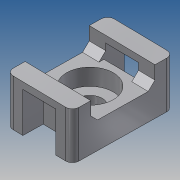
# Autodesk Inventor part: Příchytka pásků, pro M3, přírodní bílá
Saved by Autodesk Inventor 2020.4 (Build 244396000, 396)
## iProperties
Created: 2021-11-17
Part Number: Příchytka pásků, pro M3, přírodní bílá
Material: Plast, neprůhledný bílý
Catalog Web Link: https://www.plastovesoucastky.cz/cs/c/prichytky-pasku/prichytky-pasku-116?rozmerA=3.4
Vendor: plastovesoucastky
Document SubType Name: Modeling
Designer: Jiří Kizek
Manufacturer: Standard
Standards Organization: Custom
Mass: 0.453772 g
Surface Area: 7.13317 cm^2
Volume: 0.476652 cm^3
Density: 0.952 g/cm^3
Appearance: Hladká – bílá
Title: Příchytka pásků, pro M3, přírodní bílá
Author: Jiří Kizek
Keywords: 116 0004 000 02
QRDstProp: ███████ █████ ███████ █     █ █ █ █ █     █ █ ███ █ █     █ ███ █ █ ███ █ ████  █ ███ █ █ ███ █     █ █ ███ █ █     █ ██ █  █     █ ███████ █ █ █ ███████          ████         ██  ███  █ █   █ ████ █ █ ██ █   ██  █ █ ██  ██   ███ ██  █████   ██  ██ █ ██  ██ █ █   ██████████  ███   ██          ██  ███   ███ ███████  ██ ██     ██ █     █ █  ██  █ █    █ ███ █ ██ █  ███████ █ ███ █    ██  █ █ ██ █ ███ █   ██  █████   █     █ █    ██ █ █ █ ███████ ██  ███   ███
QRSrcProp: =<Part number> <Revision Number>
Povrch: 7,1331712703259
Hmotnost: 0,453772439604439
ProduktSkupina: 530
Autodesk Inventor part; units mm, degrees
ref_plane "YZ Plane" through (0, 0, 0) normal (1, 0, 0) x (0, 1, 0)
ref_plane "XZ Plane" through (0, 0, 0) normal (0, 1, 0) x (-1, 0, 0)
ref_plane "XY Plane" through (0, 0, 0) normal (0, 0, 1) x (1, 0, 0)
sketch "Náčrt6" plane through (0, 0, 0) normal (0, 1, 0) x (-1, 0, 0)
  line L0 (-7.5, 5) -> (7.5, 5)
  line L1 (7.5, 5) -> (7.5, -5)
  line L2 (7.5, -5) -> (-7.5, -5)
  line L3 (-7.5, -5) -> (-7.5, 5)
  line L4 (-7.5, 5) -> (7.5, -5) construction
  line L5 (7.5, 5) -> (-7.5, -5) construction
  point P0 (0, 0)
  dimension "d10" = 15
  dimension "d11" = 10
  constraints: 12 end point, 2 midpoint, 2 parallel, 1 horizontal, 1 perpendicular
  measures "d10" distance of L1.end L2.end
  measures "d11" distance of L0.end L1.end
extrude "Vysunutí6" add sketch "Náčrt6" along normal blind 7
sketch "Náčrt7" plane through (0, 0, 0) normal (0, 0, 1) x (1, 0, 0)
  line L0 (0, 8.4) -> (0, -1.4) projected
  line L1 (-10.5, 0) -> (10.5, 0) projected
  line L2 (-4.75, 7) -> (4.75, 7)
  line L3 (4.75, 7) -> (4.75, 5)
  line L4 (3.75, 4) -> (-3.75, 4)
  line L5 (-4.75, 5) -> (-4.75, 7)
  line L6 (7.5, 7) -> (-7.5, 7) projected
  line L7 (-4.75, 5) -> (-3.75, 4)
  line L8 (3.75, 4) -> (4.75, 5)
  point P0 (0, 0)
  point P1 (4.75, 4)
  point P2 (-4.75, 4)
  dimension "d14" = 9.5
  dimension "d15" = 3
  dimension "d16" = 1
  dimension "d17" = 1
  dimension "d18" = 1
  dimension "d19" = 1
  constraints: 12 end point, 4 point on line, 2 parallel, 1 collinear, 1 horizontal, 1 perpendicular, 1 other
  measures "d14" distance of point (4.75, 4) point (-4.75, 4)
  measures "d15" distance of L2.end point (4.75, 4)
  measures "d16" distance of L5.start point (-4.75, 4)
  measures "d17" distance of L4.end point (-4.75, 4)
  measures "d18" distance of L4.start point (4.75, 4)
  measures "d19" distance of L3.end point (4.75, 4)
extrude "Vysunutí7" cut sketch "Náčrt7" against normal through all both and the other way through all
sketch "Náčrt8" plane through (7.5, 0, 5) normal (1, 0, 0) x (0, 0, -1)
  line L0 (0, 0) -> (10, 0) projected
  line L1 (2.5, 0) -> (7.5, 0)
  line L2 (7.5, 0) -> (7.5, 6)
  line L3 (7.5, 6) -> (2.5, 6)
  line L4 (2.5, 6) -> (2.5, 0)
  line L5 (-2, 0) -> (12, 0) projected
  line L6 (5, -1.4) -> (5, 8.4) projected
  point P0 (5, 0)
  dimension "d22" = 5
  dimension "d23" = 6
  constraints: 8 end point, 2 parallel, 1 horizontal, 1 perpendicular, 1 point on line, 1 symmetric about line
  measures "d22" distance of L2.end L3.end
  measures "d23" distance of L1.end L2.end
extrude "Vysunutí8" cut sketch "Náčrt8" against normal blind 3
mirror "Zrcadlit1" about plane through (0, 0, 0) normal (1, 0, 0) of "Vysunutí8"
sketch "Náčrt9" plane through (4.5, 0, 5) normal (1, 0, 0) x (0, 0, -1)
  line L0 (2.5, 4.75) -> (7.5, 4.75) projected
  line L1 (2.5, 0) -> (2.5, 4.75) projected
  line L2 (7.5, 0) -> (2.5, 0) projected
  line L3 (7.5, 4.75) -> (7.5, 0) projected
  line L4 (10, 4) -> (0, 4) projected
  point P0 (5, 0)
  point P1 (2.5, 4)
  point P2 (7.5, 4)
extrude "Vysunutí9" cut sketch "Náčrt9" against normal through all contours L0 L3 L4 L1
sketch "Náčrt10" plane through (-3.75, 4, -5) normal (0, 1, 0) x (1, 0, 0)
  point P0 (3.75, -5)
hole "Díra1" at (0, 4, 0) direction (0, -1, 0) diameter 3.7 end through all counterbore diameter 7 counterbore depth 2.5
fillet "Zaoblení1" radius 1 4 edges at (7.5, 3.5, -5) (7.5, 3.5, 5) (-7.5, 3.5, -5) (-7.5, 3.5, 5)
equation "\"d17\" = d16"
equation "\"d18\" = d16"
equation "\"d19\" = d18"
equation "\"Milimetr\" = 1"
